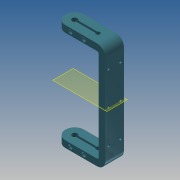
# Autodesk Inventor part: SCREW slide frame
Saved by Autodesk Inventor 2013 (Build 170138000, 138)
## iProperties
Created: 2017-03-30
Part Number: SCREW slide frame
Material: Generic
Document SubType Name: Modeling
Designer: employee
Density: 1 g/cm^3
Author: employee
Autodesk Inventor part; units mm, degrees
ref_plane "YZ Plane" through (0, 0, 0) normal (1, 0, 0) x (0, 1, 0)
ref_plane "XZ Plane" through (0, 0, 0) normal (0, 1, 0) x (-1, 0, 0)
ref_plane "XY Plane" through (0, 0, 0) normal (0, 0, 1) x (1, 0, 0)
sketch "Sketch1" plane through (0, 0, 0) normal (0, 0, 1) x (1, 0, 0)
  line L0 (0, 14) -> (60, 14)
  line L1 (60, 14) -> (60, -14)
  line L2 (60, -14) -> (0, -14)
  arc A0 (0, 14) -> (0, -14) centre (0, 0) ccw
  dimension "d0" = 60
  dimension "d2" = 28
  constraints: 6 end point, 2 point on circle, 2 tangent, 1 centre point, 1 coincident, 1 horizontal, 1 parallel, 1 perpendicular
  measures "d0" distance of L1.end L2.end
  measures "d2" distance between parallel lines of L0 L2
extrude "Extrusion1" add sketch "Sketch1" along normal blind 10
sketch "Sketch2" plane through (60, -14, 0) normal (1, 0, 0) x (0, 0, -1)
  line L0 (0, 28) -> (0, 0) projected
  line L1 (0, 28) -> (-10, 28) projected
  line L2 (0, 0) -> (-10, 0) projected
  line L3 (-10, 28) -> (150, 28)
  line L4 (150, 28) -> (150, 0)
  line L5 (150, 0) -> (-10, 0)
  line L6 (-10, 0) -> (-10, 28)
  point P0 (0, 14)
  dimension "d5" = 160
  constraints: 8 end point, 2 parallel, 1 horizontal, 1 perpendicular
  measures "d5" distance of L4.end L2.end
extrude "Extrusion2" add sketch "Sketch2" against normal blind 10 contours L3 L4 L5 L0
sketch "Sketch3" plane through (60, -14, -150) normal (0, 0, -1) x (-1, 0, 0)
  line L0 (10, 28) -> (10, 0) projected
  line L1 (10, 0) -> (60, 0) projected
  arc A0 (60, 0) -> (60, 28) centre (60, 14) ccw projected
  line L2 (60, 28) -> (10, 28) projected
extrude "Extrusion3" add sketch "Sketch3" against normal blind 10
fillet "Fillet2" radius 2.5 2 edges at (50, 0, -140) (50, 0, 0)
fillet "Fillet2" radius 12.5 2 edges at (60, 0, 10) (60, 0, -150)
sketch "Sketch11" plane through (50, -14, 0) normal (-1, 0, 0) x (0, 0, 1)
  line L0 (-140, 0) -> (-137.5, 0) projected
  line L1 (-137.5, 0) -> (-137.5, 28) projected
  line L2 (-137.5, 28) -> (-140, 28) projected
  line L3 (-140, 28) -> (-140, 0) projected
  line L4 (-120, 23) -> (-120, 5)
  line L5 (-140, 0) -> (-140, 28) projected
  circle A0 centre (-120, 23) radius 1.75
  circle A1 centre (-120, 5) radius 1.75
  point P0 (0, 14)
  point P1 (-140, 14)
  point P2 (-120, 14)
  dimension "d49" = 20
  dimension "d50" = 3.5
  dimension "d51" = 18
  constraints: 2 centre point, 2 coincident, 2 end point, 2 midpoint, 1 equal radius, 1 horizontal alignment, 1 parallel
  measures "d49" distance between parallel lines of L4 L3
  measures "d50" diameter of A0
  measures "d51" distance of L4.start L4.end
extrude "Extrusion11" cut sketch "Sketch11" against normal through all contours A0 | A1
sketch "Sketch12" plane through (50, -14, 0) normal (-1, 0, 0) x (0, 0, 1)
  circle A0 centre (-120, 23) radius 1.75 projected
  circle A1 centre (-120, 5) radius 1.75 projected
  line L0 (-123.1754, 23) -> (-121.5877, 25.75)
  line L1 (-121.5877, 25.75) -> (-118.4123, 25.75)
  line L2 (-118.4123, 25.75) -> (-116.8246, 23)
  line L3 (-116.8246, 23) -> (-118.4123, 20.25)
  line L4 (-118.4123, 20.25) -> (-121.5877, 20.25)
  line L5 (-121.5877, 20.25) -> (-123.1754, 23)
  line L6 (-123.1754, 5) -> (-121.5877, 7.75)
  line L7 (-121.5877, 7.75) -> (-118.4123, 7.75)
  line L8 (-118.4123, 7.75) -> (-116.8246, 5)
  line L9 (-116.8246, 5) -> (-118.4123, 2.25)
  line L10 (-118.4123, 2.25) -> (-121.5877, 2.25)
  line L11 (-121.5877, 2.25) -> (-123.1754, 5)
  point P0 (0, 14)
  dimension "d54" = 5.5
  constraints: 24 end point, 2 coincident, 2 horizontal, 1 parallel, 26 other
  measures "d54" distance between parallel lines of L1 L4
extrude "Extrusion12" cut sketch "Sketch12" against normal blind 4
pattern_linear "Rectangular Pattern2" count 3 spacing 50 along (0, 0, 1) of "Extrusion11", "Extrusion12"
sketch "Sketch17" plane through (0, 0, 10) normal (0, 0, 1) x (1, 0, 0)
  arc A0 (0, 14) -> (0, -14) centre (0, 0) ccw projected
  circle A1 centre (0, 0) radius 4
  circle A2 centre (35, 0) radius 3
  dimension "d79" = 8
  dimension "d81" = 6
  dimension "d82" = 35
  constraints: 2 centre point, 1 coincident, 1 horizontal alignment
  measures "d79" diameter of A1
  measures "d81" diameter of A2
  measures "d82" distance of A2.centre A0.centre
extrude "Extrusion17" cut sketch "Sketch17" against normal through all
sketch "Sketch18" plane through (0, 0, 10) normal (0, 0, 1) x (1, 0, 0)
  circle A0 centre (35, 0) radius 3 projected
  circle A1 centre (0, 0) radius 4 projected
  line L0 (0, 1.5) -> (35, 1.5)
  line L1 (35, 1.5) -> (35, -1.5)
  line L2 (35, -1.5) -> (0, -1.5)
  line L3 (0, -1.5) -> (0, 1.5)
  dimension "d85" = 3
  constraints: 8 end point, 2 coincident, 2 midpoint, 2 parallel, 1 horizontal, 1 perpendicular
  measures "d85" distance between parallel lines of L0 L2
extrude "Extrusion18" cut sketch "Sketch18" against normal through all contours L0 L1 L2 A0 | A0 L2 A1 L0 | A1 L2 L3 L0 picked at (34.0055, 0.1045) picked at (1.3333, 0)
sketch "Sketch19" plane through (0, -14, 0) normal (0, -1, 0) x (1, 0, 0)
  line L0 (0, 0) -> (0, 10) projected
  circle A0 centre (7.5, 5) radius 1.75
  circle A1 centre (27.5, 5) radius 1.75
  point P0 (0, 5)
  dimension "d89" = 27.5
  dimension "d90" = 7.5
  dimension "d91" = 3.5
  constraints: 2 centre point, 2 horizontal alignment, 1 equal radius, 1 midpoint
  measures "d89" distance from line of A1.centre L0
  measures "d90" distance from line of A0.centre L0
  measures "d91" diameter of A1
extrude "Extrusion19" cut sketch "Sketch19" against normal through all
sketch "Sketch20" plane through (0, -14, 0) normal (0, -1, 0) x (1, 0, 0)
  circle A0 centre (7.5, 5) radius 1.75 projected
  circle A1 centre (27.5, 5) radius 1.75 projected
  circle A2 centre (7.5, 5) radius 3
  circle A3 centre (27.5, 5) radius 3
  dimension "d94" = 6
  constraints: 2 centre point, 2 coincident, 1 equal radius
  measures "d94" diameter of A2
extrude "Extrusion20" cut sketch "Sketch20" against normal blind 3
sketch "Sketch21" plane through (0, 14, 10) normal (0, 1, 0) x (1, 0, 0)
  circle A0 centre (7.5, 5) radius 1.75 projected
  circle A1 centre (27.5, 5) radius 1.75 projected
  line L0 (7.5, 8.1754) -> (10.25, 6.5877)
  line L1 (10.25, 6.5877) -> (10.25, 3.4123)
  line L2 (10.25, 3.4123) -> (7.5, 1.8246)
  line L3 (7.5, 1.8246) -> (4.75, 3.4123)
  line L4 (4.75, 3.4123) -> (4.75, 6.5877)
  line L5 (4.75, 6.5877) -> (7.5, 8.1754)
  line L6 (27.5, 8.1754) -> (30.25, 6.5877)
  line L7 (30.25, 6.5877) -> (30.25, 3.4123)
  line L8 (30.25, 3.4123) -> (27.5, 1.8246)
  line L9 (27.5, 1.8246) -> (24.75, 3.4123)
  line L10 (24.75, 3.4123) -> (24.75, 6.5877)
  line L11 (24.75, 6.5877) -> (27.5, 8.1754)
  dimension "d98" = 5.5
  constraints: 24 end point, 2 coincident, 2 vertical, 1 parallel, 26 other
  measures "d98" distance between parallel lines of L7 L10
extrude "Extrusion21" cut sketch "Sketch21" against normal blind 4
ref_plane "Work Plane2" through (0, 0, -70) normal (0, 0, 1) x (1, 0, 0)
mirror "Mirror1" about plane through (0, 0, -70) normal (0, 0, 1) of "Extrusion21", "Extrusion20", "Extrusion19"
body "Solid1"
